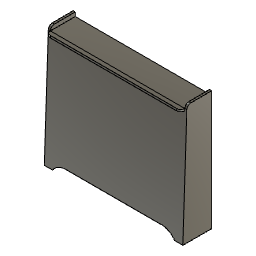
model (Autodesk Fusion 360 design; units mm, degrees)
Autodesk Fusion 360 part; units mm, degrees
sketch "Sketch1" plane through (0, 0, 0) normal (1, 0, 0) x (0, 1, 0) in component "box"
  line L0 (0, 0) -> (250, 0)
  line L1 (250, 0) -> (250, 350)
  line L2 (250, 350) -> (0, 350)
  line L3 (0, 350) -> (0, 0) construction
  line L4 (0, 350) -> (0, 368)
  line L5 (0, 368) -> (268, 368)
  line L6 (268, 368) -> (268, -18)
  line L7 (268, -18) -> (0, -18)
  line L8 (0, -18) -> (0, 0)
  line L9 (125, 350) -> (125, 368) construction
  line L10 (250, 175) -> (268, 175) construction
  line L11 (125, 0) -> (125, -18) construction
  dimension "d8" = 350
  dimension "d9" = 250
  dimension "d10" = 18
  constraint horizontal L0
  constraint vertical L1
  constraint horizontal L2
  constraint vertical L3
  constraint coincident L0.start L3.end
  constraint vertical L4
  constraint horizontal L5
  constraint vertical L6
  constraint horizontal L7
  constraint vertical L8
  constraint midpoint L2 L9.start
  constraint coincident L5 L9.end
  constraint perpendicular L5 L9
  constraint midpoint L1 L10.start
  constraint midpoint L6 L10.end
  constraint perpendicular L6 L10
  constraint midpoint L0 L11.start
  constraint coincident L7 L11.end
  constraint perpendicular L7 L11
  constraint equal L9 L10
  measures "d8" distance of L0.end L1.end
  measures "d9" distance of L0.start L0.end
  measures "d10" distance of L7.end L0.start
extrude "Extrude1" add sketch "Sketch1" against normal blind 100 makes body 1 in component "box"
sketch "Sketch1 (2)" plane through (0, 0, 0) normal (1, 0, 0) x (0, 1, 0) in component "hinge"
  line L0 (0, 347) -> (18, 347)
  line L1 (18, 347) -> (18, 3)
  line L2 (18, 3) -> (0, 3)
  line L3 (0, 3) -> (0, 347)
  line L4 (250, 350) -> (0, 350) construction
  line L5 (0, 0) -> (250, 0) construction
  line L6 (0, 0) -> (0, 3) construction
  line L7 (0, 347) -> (0, 350) construction
  circle A0 centre (23, 103) radius 5
  circle A1 centre (23, 103) radius 102.6109 construction
  circle A2 centre (23, 103) radius 244.0512 construction
  line L8 (18, 3) -> (245.623, 3)
  line L9 (245.623, 3) -> (245.623, 12)
  line L10 (245.623, 12) -> (18, 12)
  line L11 (131.8115, 12) -> (131.8115, 203)
  line L12 (131.8115, 203) -> (122.8115, 203)
  line L13 (122.8115, 203) -> (122.8115, 12)
  line L14 (236.623, 12) -> (236.623, 203) construction
  line L15 (236.623, 203) -> (245.623, 203)
  line L16 (245.623, 203) -> (245.623, 12) construction
  line L17 (122.8115, 107.5) -> (18, 107.5) construction
  line L18 (131.8115, 107.5) -> (236.623, 107.5) construction
  circle A3 centre (23, 103) radius 222.623 construction
  line L19 (250, 0) -> (250, 350) construction
  line L20 (245.623, 203) -> (222.967, 12)
  line L21 (236.623, 203) -> (213.967, 12)
  line L22 (222.967, 12) -> (221.8995, 3)
  dimension "d13" = 3
  dimension "d14" = 18
  dimension "d16" = 10
  dimension "d17" = 5
  dimension "d18" = 100
  dimension "d24" = 9
  dimension "d27" = 191
  constraint horizontal L0
  constraint vertical L1
  constraint horizontal L2
  constraint vertical L3
  constraint coincident L5.start L6.start
  constraint coincident L4.end L7.end
  constraint vertical L7
  constraint equal L6 L7
  constraint concentric A0 A1
  constraint coincident L2.end A1
  constraint coincident L0.end A2
  constraint coincident A0.centre A1.centre
  constraint horizontal L8
  constraint vertical L9
  constraint horizontal L10
  constraint coincident L1 L10.end
  constraint vertical L11
  constraint horizontal L12
  constraint vertical L13
  constraint coincident L10 L13.end
  constraint coincident L10 L11.start
  constraint vertical L14
  constraint horizontal L15
  constraint vertical L16
  constraint coincident L10 L14.start
  constraint equal L12 L15
  constraint equal L9 L15
  constraint midpoint L13 L17.start
  constraint coincident L1 L17.end
  constraint perpendicular L1 L17
  constraint midpoint L11 L18.start
  constraint coincident L14 L18.end
  constraint perpendicular L14 L18
  constraint equal L17 L18
  constraint coincident A2 L8.end
  constraint equal L11 L14
  constraint coincident A2 L15.end
  constraint concentric A2 A3
  constraint coincident L10 L20.end
  constraint coincident L10 L21.end
  constraint parallel L20 L21
  constraint tangent L16 A3
  constraint coincident L8 L22.end
  constraint collinear L20 L22
  constraint coincident A3 L22.end
  measures "d13" distance of L0.start L4.end
  measures "d14" distance of L0.start L0.end
  measures "d16" diameter of A0
  measures "d17" horizontal distance of L1.end A0.centre
  measures "d18" vertical distance of L1.end A0.centre
  measures "d24" distance of L8.end L9.end
  measures "d27" distance of L9.end L15.end
sketch "Sketch1 (3)" plane through (0, 0, 0) normal (0, 1, 0) x (1, 0, 0) in component "rack"
  line L0 (0, 0) -> (0, -1000)
  line L1 (0, -1000) -> (1200, -1000)
  line L2 (1200, -1000) -> (1200, 0)
  line L3 (1200, 0) -> (0, 0)
  line L4 (600, -1000) -> (600, 0) construction
  arc A0 (70, 0) -> (184.8913, -60) centre (184.8913, 80) ccw
  line L5 (184.8913, -60) -> (600, -60)
  line L6 (1015.1087, -60) -> (600, -60)
  arc A1 (1015.1087, -60) -> (1130, 0) centre (1015.1087, 80) ccw
  arc A2 (70, -130) -> (1130, -130) centre (600, -130) ccw
  line L7 (70, -130) -> (1130, -130)
  line L8 (70, 0) -> (70, -1000) construction
  line L9 (70, -500) -> (0, -500) construction
  line L10 (392.4456, -60) -> (392.4456, -130) construction
  line L11 (392.4456, -930) -> (392.4456, -1000) construction
  dimension "d31" = 1000
  dimension "d32" = 1200
  dimension "d33" = 1200
  dimension "d34" = 70
  dimension "d35" = 60
  dimension "d36" = 140
  constraint coincident L0.start L3.end
  constraint horizontal L1
  constraint horizontal L3
  constraint midpoint L1 L4.start
  constraint midpoint L3 L4.end
  constraint vertical L4
  constraint coincident L3 A0.start
  constraint coincident L4 L5.end
  constraint perpendicular L4 L5
  constraint tangent A0 L5
  constraint symmetric L4 A0.start A1.end
  constraint symmetric L4 A0.end L6.start
  constraint symmetric L4 A0 A1
  constraint symmetric L4 L5.end L6.end
  constraint horizontal L7
  constraint coincident A2.centre L7
  constraint coincident L4 A2.centre
  constraint coincident L1 L8.end
  constraint parallel L0 L8
  constraint tangent A2 L8
  constraint midpoint L8 L9.start
  constraint coincident L0 L9.end
  constraint perpendicular L0 L9
  constraint midpoint L5 L10.start
  constraint coincident L7 L10.end
  constraint perpendicular L7 L10
  constraint equal L9 L10
  constraint coincident L1 L11.end
  constraint perpendicular L1 L11
  constraint collinear L10 L11
  constraint equal L10 L11
  measures "d31" distance of L1 L3
  measures "d32" distance of L2.end L0.start
  measures "d33" distance of L0.end L1.end
  measures "d34" distance of L0.start A0.start
  measures "d35" distance of L3 L5
  measures "d36" radius of A0
extrude "Extrude4" add sketch "Sketch1 (3)" along normal blind 250 separate body contours L0 L1 L2 L3 A0 L5 L6 A1 | A2 L7 makes body 2 in component "rack"
draft "Draft1" angle 2 neutral plane through (0, 0, 0) pull (0, 0, 1) 1 faces at (600, 0, 686.6667) on bodies 2 in component "rack"
sketch "Sketch3" plane through (0, 0, 0) normal (-1, 0, 0) x (0, -1, 0) in component "rack"
  line L0 (0, 0) -> (-34.9208, 1000)
  line L1 (-34.9208, 1000) -> (-250, 1000)
  line L2 (-250, 1000) -> (-250, 0)
  line L3 (-250, 0) -> (0, 0)
  arc A0 (-34.9208, 1000) -> (-69.6622, 1033.7777) centre (-69.8994, 998.7785) ccw
  line L4 (-250, 1000) -> (-250, 1035)
  line L5 (-250, 1035) -> (-69.6622, 1033.7777)
  dimension "d59" = 35
  dimension "d60" = 35
  constraint tangent L0 A0
  constraint coincident L0.end L1.start
  constraint coincident L1.end L2.start
  constraint perpendicular L1 L4
  constraint tangent A0 L5
  measures "d59" radius of A0
  measures "d60" distance of L1.end L4.end
extrude "Extrude5" add sketch "Sketch3" against normal blind 18 contours L1 A0 L4 L5 bodies 2 in component "rack"
extrude "Extrude6" add sketch "Sketch3" along normal blind 18 from surface at -1200 contours L1 A0 L4 L5 bodies 2 in component "rack"
sketch "Sketch4" plane through (0, 0, 1000) normal (0, 0, 1) x (-1, 0, 0) in component "rack"
  line L0 (-1182, -34.9208) -> (-1182, -250)
  line L1 (-1182, -250) -> (-18, -250)
  line L2 (-18, -250) -> (-18, -34.9208)
  line L3 (-18, -34.9208) -> (-1182, -34.9208)
  line L4 (0, 0) -> (-1200, 0)
  arc A0 (-18, -34.9208) -> (-52.9208, 0) centre (-52.9208, -34.9208) ccw
  line L5 (-600, 0) -> (-600, -34.9208)
  constraint tangent L2 A0
  constraint coincident L4 A0.end
  constraint coincident L2.end L3.start
  constraint tangent L4 A0
  constraint midpoint L4 L5.start
  constraint midpoint L3 L5.end
extrude "Extrude7" add sketch "Sketch4" against normal blind 18 separate body contours L3 L4 A0 L5 makes body 3 in component "rack"
mirror "Mirror1" about plane through (600, 0, 1000) normal (1, 0, 0) of bodies 3 merged in component "rack"
sketch "Sketch5" plane through (0, 0, 0) normal (0, 0, -1) x (1, 0, 0) in component "rack"
  line L0 (70, 0) -> (0, 0)
  line L1 (0, 0) -> (0, -250)
  line L2 (0, -250) -> (70, -250)
  line L3 (70, -250) -> (70, 0)
  line L4 (0, 0) -> (1200, 0) construction
  line L5 (1200, 0) -> (1200, -250) construction
  line L6 (1200, -250) -> (0, -250) construction
  line L7 (0, -250) -> (0, 0) construction
  line L8 (18, -18) -> (1182, -18)
  line L9 (1182, -18) -> (1182, -232)
  line L10 (1182, -232) -> (18, -232)
  line L11 (18, -232) -> (18, -18)
  point P0 (1200, -250)
  dimension "d70" = 18
  constraint horizontal L4
  constraint vertical L5
  constraint horizontal L6
  constraint vertical L7
  constraint coincident P0 L5.end
  constraint coincident L0.end L1.start
extrude "Extrude8" cut sketch "Sketch5" against normal up to surface (60 mm away) contours L3 L8 L9 L10 | L3 L8 L10 L11 bodies 2 in component "rack"
component "mechanism" placed x (1, 0, 0) y (0, 1, 0) z (0, 0, 1) at (0, 0, 0)
component "rack" placed x (1, 0, 0) y (0, 1, 0) z (0, 0, 1) at (0, 0, 0)
component "box" placed x (1, 0, 0) y (0, 1, 0) z (0, 0, 1) at (0, 0, 0) in component "mechanism"
component "hinge" placed x (1, 0, 0) y (0, 1, 0) z (0, 0, 1) at (0, 0, 0) in component "mechanism"
equation "d59 = d60"
